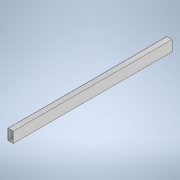
# Autodesk Inventor part: 30in OChannel 1x2
Saved by Autodesk Inventor 2020 (Build 240168000, 168)
## iProperties
Created: 2021-02-04
Part Number: 30in OChannel 1x2
Material: Aluminum 6061-AHC
Document SubType Name: Modeling
Designer: sidsa
Density: 2.7 g/cm^3
Appearance: Aluminum - Dark
Author: sidsa
Autodesk Inventor part; units mm, degrees
ref_plane "YZ Plane" through (0, 0, 0) normal (1, 0, 0) x (0, 1, 0)
ref_plane "XZ Plane" through (0, 0, 0) normal (0, 1, 0) x (-1, 0, 0)
ref_plane "XY Plane" through (0, 0, 0) normal (0, 0, 1) x (1, 0, 0)
sketch "Sketch1" plane through (0, 0, 0) normal (0, 0, 1) x (1, 0, 0)
  line L0 (0, 0) -> (25.4, 0)
  line L1 (25.4, 0) -> (25.4, 50.8)
  line L2 (25.4, 50.8) -> (0, 50.8)
  line L3 (0, 50.8) -> (0, 0)
  line L4 (24.384, 49.784) -> (24.384, 1.016)
  line L5 (24.384, 1.016) -> (1.016, 1.016)
  line L6 (1.016, 1.016) -> (1.016, 49.784)
  line L7 (1.016, 49.784) -> (24.384, 49.784)
  dimension "d0" = 25.4
  dimension "d1" = 50.8
  dimension "d2" = 1.016
  constraints: 16 end point, 4 parallel, 2 perpendicular, 1 horizontal, 3 other
  measures "d0" distance of L2.end L1.end
  measures "d1" distance of L0.end L1.end
  measures "d2" distance between parallel lines of L1 L4
extrude "Extrusion1" add sketch "Sketch1" along normal blind 762
body "Solid1"
